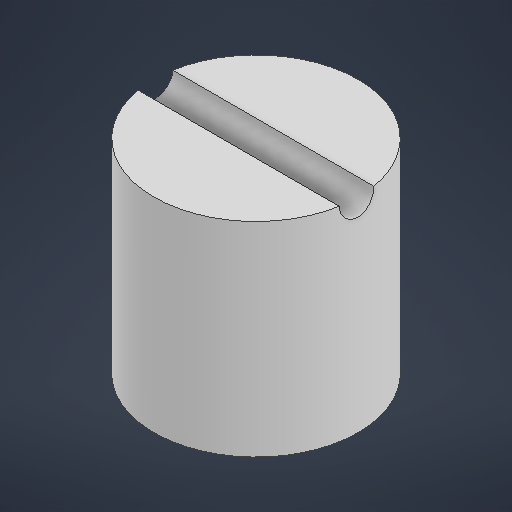
# Autodesk Inventor part: rodamiento
Saved by Autodesk Inventor 2025.3 (Build 293356000, 356)
## iProperties
Created: 2025-10-02
Part Number: rodamiento
Material: Generic
Document SubType Name: Modeling
Designer: sophi
Density: 1 g/cm^3
Appearance: Default
Author: sophi
Autodesk Inventor part; units mm, degrees
ref_plane "YZ Plane" through (0, 0, 0) normal (1, 0, 0) x (0, 1, 0)
ref_plane "XZ Plane" through (0, 0, 0) normal (0, 1, 0) x (-1, 0, 0)
ref_plane "XY Plane" through (0, 0, 0) normal (0, 0, 1) x (1, 0, 0)
sketch "Sketch1" plane through (0, 0, 0) normal (0, 1, 0) x (-1, 0, 0)
  circle A0 centre (0, 0) radius 5
  circle A1 centre (0, 0) radius 4.25
  dimension "d0" = 10
  dimension "d1" = 8.5
  constraints: 2 centre point, 2 coincident
  measures "d0" diameter of A0
  measures "d1" diameter of A1
extrude "Extrusion1" add sketch "Sketch1" along normal blind 10 contours A0 | A1
extrude "Extrusion2" cut sketch "Sketch1" along normal blind 5 contours A1
sketch "Sketch3" plane through (0, 0, 0) normal (1, 0, 0) x (0, 1, 0)
  circle A0 centre (10, 0) radius 0.85
  line L0 (0, -5) -> (10, -5) projected
  line L1 (0, 5) -> (10, 5) projected
  line L2 (10, -5) -> (10, 5) projected
  point P0 (0, 0)
  point P1 (10, -0.85)
  point P2 (10, 0.85)
  dimension "d9" = 1.7
  dimension "d10" = 5
  constraints: 1 centre point, 1 midpoint
  measures "d9" diameter of A0
  measures "d10" distance from line of L1 A0.centre
extrude "Extrusion4" cut sketch "Sketch3" along normal mid plane 10 contours L2 A0 picked at (9.5995, 0.1005)
body "Solid1"
